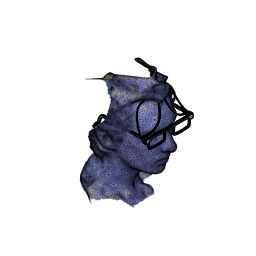
limelight_ (Autodesk Fusion 360 design; units mm, degrees)
Autodesk Fusion 360 part; units mm, degrees
note: some values were not read from the file. Set by a fixed rule: which sketch regions a step uses.
other "Base Mesh Feature1"
other "Scale1"
other "Modify1"
other "Scale2"
other "Modify2"
other "Scale3"
other "Modify3"
other "Modify4"
other "Base Mesh Feature2"
sketch "Sketch1" plane through (0, 0, 0) normal (1, 0, 0) x (0, 1, 0)
  line L0 (140.8479, 83.3353, 750) -> (440.7975, 83.3353, 750)
  line L1 (-324.1521, 83.3346, 750) -> (-324.1521, 110, 750)
  line L2 (-324.1521, 110, 750) -> (366, 110, 750)
  line L3 (440.7975, 83.3353, 750) -> (440.7975, 110, 750)
  line L4 (440.7975, 110, 750) -> (440.7975, 109, 750)
  arc A0 through (141.443, 83.3353, 750) (130.2389, 4.5049, 750) (140.8479, -74.4077, 750)
  arc A1 through (440.7975, -74.4077, 750) (453.6261, 4.4638, 750) (440.7975, 83.3353, 750)
  arc A2 through (140.8479, -74.4077, 750) (290.8227, -88.3663, 750) (440.7975, -74.4077, 750)
  line L5 (440.7975, 110, 750) -> (506.8968, 110, 750)
  line L6 (506.8968, 110, 750) -> (506.8968, 36.4474, 750)
  line L7 (506.8968, 36.4474, 750) -> (451.5624, 36.4474, 750)
  line L8 (-389.1, 110, 750) -> (-324.1521, 110, 750)
  line L9 (-389.1, 110.5472, 750) -> (-389.1, 36.4474, 750)
  line L10 (-334.8263, 36.5791, 750) -> (-389.1, 36.5791, 750)
  line L11 (366, 110, 750) -> (440.7975, 110, 750)
  line L12 (-324.1521, 83.3337, 750) -> (-324.1525, 83.3335, 750)
  line L13 (-24.2821, 83.3353, 750) -> (-324.2317, 83.3353, 750)
  arc A3 through (-324.2317, -74.4077, 750) (-337.0603, 4.4638, 750) (-324.2317, 83.3353, 750)
  arc A4 through (-24.2821, -74.4077, 750) (-174.2569, -88.3663, 750) (-324.2317, -74.4077, 750)
  arc A5 through (-24.8772, 83.3353, 750) (-13.6732, 4.5049, 750) (-24.2821, -74.4077, 750)
  line L14 (-24.8772, 83.3353, 750) -> (140.85, 83.3353, 750)
  arc A6 through (57.5187, -332.9413, 750) (68.7228, -411.7717, 750) (58.1138, -490.6843, 750)
  arc A7 through (58.1138, -490.6843, 750) (-91.861, -504.6429, 750) (-241.8358, -490.6843, 750)
  arc A8 through (-241.8358, -490.6843, 750) (-254.6644, -411.8128, 750) (-241.8358, -332.9413, 750)
  line L15 (58.1138, -332.9413, 750) -> (-241.8358, -332.9413, 750)
  line L16 (178.822, -332.9413, 750) -> (478.7716, -332.9413, 750)
  arc A9 through (179.4171, -332.9413, 750) (168.2131, -411.7717, 750) (178.822, -490.6843, 750)
  arc A10 through (178.822, -490.6843, 750) (328.7968, -504.6429, 750) (478.7716, -490.6843, 750)
  arc A11 through (478.7716, -490.6843, 750) (491.6002, -411.8128, 750) (478.7716, -332.9413, 750)
sketch "Sketch2" plane through (0, 0, 0) normal (1, 0, 0) x (0, 1, 0)
sketch "Sketch3" plane through (0, 0, 0) normal (0, 1, 0) x (1, 0, 0)
  line L0 (749.7214, -109.6566, 525) -> (-225, -109.6566, 525)
  line L1 (-225, -109.6566, 525) -> (-225, -75, 525)
  line L2 (-225, -75, 525) -> (750, -75, 525)
  line L3 (-225, -109.6566, 525) -> (-290.5465, -40.2965, 525)
  spline S0 degree 5 poles (-225, -109.6566, 525) (-229.9167, -109.8552, 525) (-239.5326, -109.7558, 525) (-253.3037, -108.1171, 525) (-270.3378, -102.903, 525) (-289.2972, -91.0605, 525) (-305.7958, -73.6023, 525) (-319.8038, -50.4603, 525) (-331.4877, -22.0144, 525) (-341.0832, 11.1976, 525) (-348.8293, 48.63, 525) (-353.7, 81.6023, 525) (-356.6609, 107.9114, 525) (-358.3321, 126.1414, 525) (-359.092, 135.4291, 525) knots 0 0 0 0 0 0 0.1 0.2 0.3 0.4 0.5 0.6 0.7 0.8 0.9 1 1 1 1 1 1
  spline S1 degree 5 poles (-225, -75, 525) (-228.9423, -74.8757, 525) (-236.6483, -74.1359, 525) (-247.6718, -71.5529, 525) (-261.2801, -65.1118, 525) (-276.384, -51.8165, 525) (-289.4959, -33.0418, 525) (-300.645, -8.8683, 525) (-309.999, 20.2425, 525) (-317.7601, 53.7351, 525) (-324.1234, 91.0724, 525) (-328.2167, 123.6855, 525) (-330.7671, 149.5743, 525) (-332.2403, 167.4582, 525) (-332.9201, 176.5564, 525) knots 0 0 0 0 0 0 0.1 0.2 0.3 0.4 0.5 0.6 0.7 0.8 0.9 1 1 1 1 1 1
  line L4 (-359.092, 135.4291, 525) -> (-332.9201, 176.5564, 525)
  line L5 (749.6084, -109.6566, 525) -> (749.6084, -75, 525)
  point P0 (-303.0094, -74.9766)
  point P1 (-283.692, -40.2965)
sketch "Sketch1 (curves 750 mm off its plane)" plane through (750, 0, 0) normal (1, 0, 0) x (0, 1, 0)
  line L0 (140.8479, 83.3353) -> (440.7975, 83.3353)
  line L1 (-324.1521, 83.3346) -> (-324.1521, 110)
  line L2 (-324.1521, 110) -> (366, 110)
  line L3 (440.7975, 83.3353) -> (440.7975, 110)
  line L4 (440.7975, 110) -> (440.7975, 109)
  arc A0 (141.443, 83.3353) -> (140.8479, -74.4077) centre (420.8756, 3.4085) ccw
  arc A1 (440.7975, -74.4077) -> (440.7975, 83.3353) centre (204.757, 4.4638) ccw
  arc A2 (140.8479, -74.4077) -> (440.7975, -74.4077) centre (290.8227, 724.3) ccw
  line L5 (440.7975, 110) -> (506.8968, 110)
  line L6 (506.8968, 110) -> (506.8968, 36.4474)
  line L7 (506.8968, 36.4474) -> (451.5624, 36.4474)
  line L8 (-389.1, 110) -> (-324.1521, 110)
  line L9 (-389.1, 110.5472) -> (-389.1, 36.4474)
  line L10 (-334.8263, 36.5791) -> (-389.1, 36.5791)
  line L11 (366, 110) -> (440.7975, 110)
  line L12 (-324.1521, 83.3337) -> (-324.1525, 83.3335)
  line L13 (-24.2821, 83.3353) -> (-324.2317, 83.3353)
  arc A3 (-324.2317, -74.4077) -> (-324.2317, 83.3353) centre (-88.1912, 4.4638) cw
  arc A4 (-24.2821, -74.4077) -> (-324.2317, -74.4077) centre (-174.2569, 724.3) cw
  arc A5 (-24.8772, 83.3353) -> (-24.2821, -74.4077) centre (-304.3099, 3.4085) cw
  line L14 (-24.8772, 83.3353) -> (140.85, 83.3353)
  arc A6 (57.5187, -332.9413) -> (58.1138, -490.6843) centre (-221.9139, -412.8681) cw
  arc A7 (58.1138, -490.6843) -> (-241.8358, -490.6843) centre (-91.861, 308.0234) cw
  arc A8 (-241.8358, -490.6843) -> (-241.8358, -332.9413) centre (-5.7953, -411.8128) cw
  line L15 (58.1138, -332.9413) -> (-241.8358, -332.9413)
  line L16 (178.822, -332.9413) -> (478.7716, -332.9413)
  arc A9 (179.4171, -332.9413) -> (178.822, -490.6843) centre (458.8497, -412.8681) ccw
  arc A10 (178.822, -490.6843) -> (478.7716, -490.6843) centre (328.7968, 308.0234) ccw
  arc A11 (478.7716, -490.6843) -> (478.7716, -332.9413) centre (242.7311, -411.8128) ccw
extrude "Extrude1" add sketch "Sketch1 (curves 750 mm off its plane)" against normal blind 25 contours L0 L1 L2 L3 L4 L11 L13 L14 | L0 A0 A1 A2 | L13 A3 A4 A5 | L3 L4 A1 L5 L6 L7 | L1 L8 L9 L10 L13 A3 makes body 1
sketch "Sketch3 (curves 525 mm off its plane)" plane through (0, 525, 0) normal (0, 1, 0) x (1, 0, 0)
  line L0 (749.7214, -109.6566) -> (-225, -109.6566)
  line L1 (-225, -109.6566) -> (-225, -75)
  line L2 (-225, -75) -> (750, -75)
  line L3 (-225, -109.6566) -> (-290.5465, -40.2965)
  spline S0 degree 5 poles (-225, -109.6566) (-229.9167, -109.8552) (-239.5326, -109.7558) (-253.3037, -108.1171) (-270.3378, -102.903) (-289.2972, -91.0605) (-305.7958, -73.6023) (-319.8038, -50.4603) (-331.4877, -22.0144) (-341.0832, 11.1976) (-348.8293, 48.63) (-353.7, 81.6023) (-356.6609, 107.9114) (-358.3321, 126.1414) (-359.092, 135.4291) knots 0 0 0 0 0 0 0.1 0.2 0.3 0.4 0.5 0.6 0.7 0.8 0.9 1 1 1 1 1 1
  spline S1 degree 5 poles (-225, -75) (-228.9423, -74.8757) (-236.6483, -74.1359) (-247.6718, -71.5529) (-261.2801, -65.1118) (-276.384, -51.8165) (-289.4959, -33.0418) (-300.645, -8.8683) (-309.999, 20.2425) (-317.7601, 53.7351) (-324.1234, 91.0724) (-328.2167, 123.6855) (-330.7671, 149.5743) (-332.2403, 167.4582) (-332.9201, 176.5564) knots 0 0 0 0 0 0 0.1 0.2 0.3 0.4 0.5 0.6 0.7 0.8 0.9 1 1 1 1 1 1
  line L4 (-359.092, 135.4291) -> (-332.9201, 176.5564)
  line L5 (749.6084, -109.6566) -> (749.6084, -75)
extrude "Extrude2" add sketch "Sketch3 (curves 525 mm off its plane)" along normal blind 20 separate body makes body 2
copy_body "CopyPasteBodies1" bodies 2 makes body 3
move_body "Move1" bodies 3 to x (1, 0, 0) y (0, 1, 0) z (0, 0, 1) at (0, -950, 0)
move_body "Move2" bodies 1 to x (1, 0, 0) y (0, 1, 0) z (0, 0, 1) at (50, 0, 0)
move_body "Move3" bodies 2 to x (1, 0, 0) y (0, 1, 0) z (0, 0, 1) at (100, 0, 0)
move_body "Move4" bodies 2 to x (1, 0, 0) y (0, 1, 0) z (0, 0, 1) at (-50, 0, 0)
extrude "Extrude3" add sketch "Sketch1 (curves 750 mm off its plane)" along normal blind 20 separate body contours A6 A7 A8 L15 | L16 A9 A10 A11 makes body 4 at (750, -108.8086, -389.6569) makes body 5 at (750, 345.7444, -389.6569)
scale "Scale1'" factor 0.9 about (770, 57.5187, -332.9413) bodies 4 5
move_body "Move5" bodies 4 to x (1, 0, 0) y (0, 1, 0) z (0, 0, 1) at (0, -100.648, 411.847)
move_body "Move6" bodies 5 to x (1, 0, 0) y (0, 1, 0) z (0, 0, 1) at (-50, -6.9412, 414.1607)
move_body "Move7" bodies 4 to x (1, 0, 0) y (0, 1, 0) z (0, 0, 1) at (-50, 0, 0)
move_body "Move8" bodies 5 to x (1, 0, 0) y (0, 1, 0) z (0, 0, 1) at (0, -0.8429, -2.0422)
extrude "Extrude4" cut 2 faces at (720, 309.1377, 28.1332) (720, -192.8239, 27.8617) along direction (1, 0, 0) blind 220 on bodies 4 5 bodies 1
other "Scale4"
other "Modify5"
other "Scale5"
other "Modify6"
other "Scale6"
other "Scale7"
scale "Scale2'" factor 0.2 about (-225, -405, 109.6566) bodies 3 1 2
move_body "Move9" bodies 3 1 2 to x (1, 0, 0) y (0, 1, 0) z (0, 0, 1) at (125, 283.3936, -86.4445)
scale "Scale3'" factor 0.7 about (-90, 68.3936, 23.2122) bodies 2 1 3
move_body "Move10" bodies 1 2 3 to x (1, 0, 0) y (0, 1, 0) z (0, 0, 1) at (40, -35, -5)
move_face "OffsetFaces1" offset -30 2 faces at (86.4452, 32.4603, 14.9776) (79.4452, -100.5397, 14.9776) on bodies 2 3
fillet "Fillet1" radius 2.25 2 edges at (84.75, -46.3059, -7.5568) (84.75, -23.1877, -7.5568) on bodies 1
fillet "Fillet2" radius 0.1 12 edges at (86.5, -1.4641, -9.5087) (86.5, -22.9109, -7.239) (86.5, -24.6634, 4.2315) (86.5, -44.8302, 4.2315) (86.5, -46.5826, -7.239) (86.5, -68.0294, -9.5087) (83, -68.0294, -9.5087) (83, -46.5826, -7.239) (83, -44.8302, 4.2315) (83, -24.6634, 4.2315) (83, -22.9109, -7.239) (83, -1.4641, -9.5087) on bodies 1
sketch "Sketch4" plane through (0, 0, 0) normal (1, 0, 0) x (0, 1, 0)
  line L0 (28.0614, 18.257, 83) -> (28.0614, 8, 83)
  line L1 (28.0614, 8, 83) -> (20.3595, 8, 83)
  arc A0 through (20.3595, 8, 83) (20.4148, 11.2668, 83) (19.1998, 14.2997, 83)
  arc A1 through (19.1998, 14.5242, 83) (19.1663, 14.4119, 83) (19.1998, 14.2997, 83)
  line L2 (19.1998, 14.5242, 83) -> (19.1998, 18.2279, 83)
  line L3 (19.1998, 18.2279, 83) -> (28.0614, 18.257, 83)
  line L4 (-88.4567, 18.1832, 82.9817) -> (-97.3183, 18.2123, 82.9817)
  line L5 (-88.4567, 14.4795, 82.9817) -> (-88.4567, 18.1832, 82.9817)
  arc A2 through (-89.6164, 7.9553, 82.9817) (-89.6717, 11.2221, 82.9817) (-88.4567, 14.255, 82.9817)
  line L6 (-97.3183, 7.9553, 82.9817) -> (-89.6164, 7.9553, 82.9817)
  line L7 (-97.3183, 18.2123, 82.9817) -> (-97.3183, 7.9553, 82.9817)
  line L8 (-88.4567, 14.4808, 82.9817) -> (-88.4567, 14.255, 82.9817)
sketch "Sketch4 (curves 82.9817 mm off its plane)" plane through (82.9817, 0, 0) normal (1, 0, 0) x (0, 1, 0)
  line L0 (-88.4567, 18.1832) -> (-97.3183, 18.2123)
  line L1 (-88.4567, 14.4795) -> (-88.4567, 18.1832)
  arc A0 (-89.6164, 7.9553) -> (-88.4567, 14.255) centre (-81.5439, 9.7258) cw
  line L2 (-97.3183, 7.9553) -> (-89.6164, 7.9553)
  line L3 (-97.3183, 18.2123) -> (-97.3183, 7.9553)
  line L4 (-88.4567, 14.4808) -> (-88.4567, 14.255)
extrude "Extrude5" add sketch "Sketch4 (curves 82.9817 mm off its plane)" against normal blind 8 separate body makes body 6
sketch "Sketch4 (curves 83 mm off its plane)" plane through (83, 0, 0) normal (1, 0, 0) x (0, 1, 0)
  line L0 (28.0614, 18.257) -> (28.0614, 8)
  line L1 (28.0614, 8) -> (20.3595, 8)
  arc A0 (20.3595, 8) -> (19.1998, 14.2997) centre (12.287, 9.7705) ccw
  arc A1 (19.1998, 14.5242) -> (19.1998, 14.2997) centre (19.3711, 14.4119) ccw
  line L2 (19.1998, 14.5242) -> (19.1998, 18.2279)
  line L3 (19.1998, 18.2279) -> (28.0614, 18.257)
extrude "Extrude6" add sketch "Sketch4 (curves 83 mm off its plane)" against normal blind 8 separate body makes body 7
sketch "Sketch5" plane through (0, 0, 0) normal (1, 0, 0) x (0, 1, 0)
  line L0 (27.0584, 11.8394, 75) -> (23.6584, 11.8394, 75)
  line L1 (23.6584, 11.8394, 75) -> (23.6584, 17.2394, 75)
  line L2 (23.6584, 17.2394, 75) -> (27.0584, 17.2394, 75)
  line L3 (27.0584, 17.2394, 75) -> (27.0584, 11.8394, 75)
  line L4 (27.0584, 11.8394, 75) -> (23.6584, 17.2394, 75) construction
  line L5 (23.6584, 11.8394, 75) -> (27.0584, 17.2394, 75) construction
  line L6 (-92.9416, 17.2394, 74.98) -> (-92.9416, 11.8394, 74.98)
  line L7 (-92.9416, 11.8394, 74.98) -> (-96.3416, 11.8394, 74.98)
  line L8 (-96.3416, 17.2394, 74.98) -> (-92.9416, 17.2394, 74.98)
  line L9 (-96.3416, 11.8394, 74.98) -> (-96.3416, 17.2394, 74.98)
  line L10 (-92.9416, 11.8394, 74.98) -> (-96.3416, 17.2394, 74.98) construction
  line L11 (-96.3416, 11.8394, 74.98) -> (-92.9416, 17.2394, 74.98) construction
  point P0 (25.3584, 14.5394)
  point P1 (-94.6416, 14.5394)
sketch "Sketch5 (curves 75 mm off its plane)" plane through (75, 0, 0) normal (1, 0, 0) x (0, 1, 0)
  line L0 (27.0584, 11.8394) -> (23.6584, 11.8394)
  line L1 (23.6584, 11.8394) -> (23.6584, 17.2394)
  line L2 (23.6584, 17.2394) -> (27.0584, 17.2394)
  line L3 (27.0584, 17.2394) -> (27.0584, 11.8394)
  line L4 (27.0584, 11.8394) -> (23.6584, 17.2394) construction
  line L5 (23.6584, 11.8394) -> (27.0584, 17.2394) construction
extrude "Extrude7" cut sketch "Sketch5 (curves 75 mm off its plane)" along normal blind 7 bodies 7
sketch "Sketch5 (curves 74.98 mm off its plane)" plane through (74.98, 0, 0) normal (1, 0, 0) x (0, 1, 0)
  line L0 (-92.9416, 17.2394) -> (-92.9416, 11.8394)
  line L1 (-92.9416, 11.8394) -> (-96.3416, 11.8394)
  line L2 (-96.3416, 17.2394) -> (-92.9416, 17.2394)
  line L3 (-96.3416, 11.8394) -> (-96.3416, 17.2394)
  line L4 (-92.9416, 11.8394) -> (-96.3416, 17.2394) construction
  line L5 (-96.3416, 11.8394) -> (-92.9416, 17.2394) construction
extrude "Extrude8" cut sketch "Sketch5 (curves 74.98 mm off its plane)" along normal blind 7 bodies 6
delete_face "DeleteFace1" 1 faces at (77.6667, 19.1945, 14.3081) on bodies 7
fillet "Fillet3" radius 0.25 12 edges at (74.9817, -97.3183, 13.0838) (74.9817, -92.8875, 18.1978) (74.9817, -88.4567, 16.2191) (74.9817, -89.6717, 11.2221) (74.9817, -93.4674, 7.9553) (78.9817, -88.4567, 14.255) (79, 19.1998, 14.2997) (75, 19.1998, 16.2638) (75, 20.4148, 11.2668) (75, 23.6306, 18.2425) (75, 28.0614, 13.1285) (75, 24.2105, 8) on bodies 6 7
fillet "Fillet4" radius 0.1 4 edges at (79.1067, -89.6164, 7.9553) (75.0383, -89.7295, 8.0469) (79.125, 20.3595, 8) (75.0566, 20.4725, 8.0916) on bodies 6 7
fillet "Fillet5" radius 0.15 4 edges at (79.1067, -88.4567, 18.1832) (75.0549, -88.5299, 18.1103) (79.125, 19.1998, 18.2279) (75.0732, 19.273, 18.155) on bodies 6 7
fillet "Fillet6" radius 0.5 8 edges at (-60.5275, 33.3936, 3.9291) (3.2226, 33.3936, 13.3602) (3.2226, 30.5936, 13.3602) (-60.5275, 30.5936, 3.9291) (-67.5275, -99.6064, 3.9291) (-3.7774, -99.6064, 13.3602) (-3.7774, -102.4064, 13.3602) (-67.5275, -102.4064, 3.9291) on bodies 2 3
move_body "Move11" bodies 2 to x (1, 0, 0) y (0, 1, 0) z (0, 0, 1) at (25, 0, 0)
move_body "Move12" bodies 3 to x (1, 0, 0) y (0, 1, 0) z (0, 0, 1) at (30, 0, 0)
move_body "Move13" bodies 1 7 6 to x (1, 0, 0) y (0, 1, 0) z (0, 0, 1) at (0, 10, 0)
sketch "Sketch6" plane through (0, 33.3936, 0) normal (0, 1, 0) x (-1, 0, 0)
  line L0 (-81.4452, 13.8602) -> (25.0079, 13.8602)
  spline S0 degree 3 poles (40.5566, -21.154) (40.2972, -17.824) (39.9613, -14.4995) (39.1496, -8.5924) (38.7212, -6.0065) (37.6122, -0.8835) (36.9383, 1.6625) (35.994, 4.1092) (35.5897, 5.1566) (35.1338, 6.1847) (33.7486, 8.7534) (32.6897, 10.2436) (30.2327, 12.3629) (28.9376, 13.0817) (26.7221, 13.7092) (25.8698, 13.8331) (25.0158, 13.86) (25.0131, 13.8601) (25.0105, 13.8602) (25.0079, 13.8602) knots -4.142023 -4.142023 -4.142023 -4.142023 -3.14001 -3.14001 -2.35323 -2.35323 -1.566445 -1.566445 -1.566445 -1.229621 -1.229621 -0.690703 -0.690703 -0.256348 -0.256348 0 0 0 0.000788 0.000788 0.000788 0.000788
  line L1 (40.5566, -21.154) -> (43.7729, -16.0998)
  spline S1 degree 5 poles (43.7729, -16.0998) (43.6665, -14.7996) (43.4325, -12.2473) (43.018, -8.5641) (42.3361, -3.948) (41.2516, 1.2926) (39.9083, 5.9423) (38.2725, 9.9247) (36.3114, 13.1646) (34.0016, 15.6087) (31.3473, 17.2667) (28.9625, 17.9966) (27.0346, 18.2261) (25.6883, 18.24) (25, 18.2122) knots -1 -1 -1 -1 -1 -1 -0.9 -0.8 -0.7 -0.6 -0.5 -0.4 -0.3 -0.2 -0.1 0 0 0 0 0 0
  line L2 (25, 18.2122) -> (-81.4452, 18.2122)
  line L3 (-81.4452, 18.2122) -> (-81.4452, 13.8602)
  spline S2 degree 5 poles (42.7082, -6.7221) (43.0306, -6.6571) (43.6683, -6.5541) (44.6034, -6.4806) (45.8069, -6.5473) (47.2345, -6.922) (48.5801, -7.6082) (49.8395, -8.6212) (51.0149, -9.9531) (52.1131, -11.5781) (53.1417, -13.4672) (53.9142, -15.1695) (54.4672, -16.5465) (54.8243, -17.5082) (55, -18) knots 0 0 0 0 0 0 0.1 0.2 0.3 0.4 0.5 0.6 0.7 0.8 0.9 1 1 1 1 1 1
  spline S3 degree 5 poles (42.988, -8.7008) (43.2023, -8.5839) (43.6304, -8.3839) (44.2715, -8.1857) (45.124, -8.1282) (46.1856, -8.4193) (47.243, -9.0924) (48.2962, -10.1488) (49.3454, -11.5605) (50.3911, -13.2902) (51.4337, -15.3007) (52.2656, -17.1101) (52.8883, -18.572) (53.303, -19.5925) (53.5102, -20.1142) knots 0 0 0 0 0 0 0.1 0.2 0.3 0.4 0.5 0.6 0.7 0.8 0.9 1 1 1 1 1 1
  line L4 (53.5102, -20.1142) -> (55, -18)
  circle A0 centre (55, -20) radius 2.1213
  point P0 (49, -8)
  point P1 (47, -9)
  constraint coincident S1 S2.start
  constraint coincident S1 S3.start
extrude "Extrude9" add sketch "Sketch6" against normal blind 3 separate body contours S1 S2 S3 A0 | S2 S3 L4 A0 | S2 S3 L4 A0 makes body 8
copy_body "CopyPasteBodies2" bodies 8 makes body 9
move_body "Move14" bodies 9 to x (1, 0, 0) y (0, 1, 0) z (0, 0, 1) at (0, -133, 0)
move_body "Move15" bodies 2 8 to x (1, 0, 0) y (0, 1, 0) z (0, 0, 1) at (0.8147, 3.352, -1.2314)
move_body "Move16" bodies 3 9 to x (1, 0, 0) y (0, 1, 0) z (0, 0, 1) at (-0.3292, 16.5, -0.9443)
sketch "Sketch7" plane through (0, 0, 16.9808) normal (0, 0, 1) x (-1, 0, 0)
  line L0 (24.1853, -33.9456) -> (-82.2599, -33.9456)
  line L1 (-82.2599, -33.9456) -> (-82.2599, -36.7456)
  line L2 (-82.2599, -36.7456) -> (24.1853, -36.7456)
  line L3 (24.1853, -36.7456) -> (24.1853, -33.9456)
  line L4 (-58.886, -33.9456) -> (-52.6505, -33.9456)
  line L5 (-52.6505, -33.9456) -> (-52.6505, -36.7456)
  line L6 (-52.6505, -36.7456) -> (-58.886, -36.7456)
  line L7 (-58.886, -36.7456) -> (-58.886, -33.9456)
  constraint horizontal L4
  constraint vertical L5
  constraint horizontal L6
  constraint vertical L7
  constraint coincident L2 L5.end
  constraint coincident L0 L4.start
sketch "Sketch8" plane through (0, 36.7456, 0) normal (0, 1, 0) x (-1, 0, 0)
  line L0 (-82.2599, 12.6288) -> (24.1931, 12.6288)
  spline S0 degree 3 poles (39.7418, -22.3854) (39.4825, -19.0554) (39.1466, -15.7309) (38.3348, -9.8238) (37.9065, -7.2379) (36.7974, -2.1149) (36.1236, 0.4311) (35.1792, 2.8778) (34.7749, 3.9252) (34.3191, 4.9533) (32.9339, 7.522) (31.875, 9.0122) (29.418, 11.1315) (28.1229, 11.8503) (25.9073, 12.4778) (25.0551, 12.6017) (24.201, 12.6286) (24.1984, 12.6287) (24.1958, 12.6288) (24.1931, 12.6288) knots -4.142023 -4.142023 -4.142023 -4.142023 -3.14001 -3.14001 -2.35323 -2.35323 -1.566445 -1.566445 -1.566445 -1.229621 -1.229621 -0.690703 -0.690703 -0.256348 -0.256348 0 0 0 0.000788 0.000788 0.000788 0.000788
  line L1 (39.7418, -22.3854) -> (42.9581, -17.3312)
  spline S1 degree 5 poles (42.9581, -17.3312) (42.8518, -16.031) (42.6178, -13.4787) (42.2033, -9.7955) (41.5214, -5.1794) (40.4369, 0.0612) (39.0935, 4.7109) (37.4578, 8.6933) (35.4967, 11.9332) (33.1869, 14.3773) (30.5326, 16.0353) (28.1478, 16.7652) (26.2198, 16.9947) (24.8736, 17.0086) (24.1853, 16.9808) knots -1 -1 -1 -1 -1 -1 -0.9 -0.8 -0.7 -0.6 -0.5 -0.4 -0.3 -0.2 -0.1 0 0 0 0 0 0
  line L2 (24.1853, 16.9808) -> (-82.2599, 16.9808)
  line L3 (-82.2599, 16.9808) -> (-82.2599, 12.6288)
  spline S2 degree 5 poles (-56, 19) (-56.5276, 20.0173) (-57.5618, 22.0263) (-59.0501, 24.9632) (-60.9065, 28.7234) (-62.9962, 33.1433) (-64.8263, 37.2476) (-66.359, 40.9905) (-67.5538, 44.3228) (-68.3753, 47.2013) (-68.8111, 49.611) (-68.8621, 51.1771) (-68.7404, 52.1573) (-68.5894, 52.7258) (-68.4965, 52.9889) knots 0 0 0 0 0 0 0.1 0.2 0.3 0.4 0.5 0.6 0.7 0.8 0.9 1 1 1 1 1 1
  point P0 (-68, 46)
sketch "Sketch9" plane through (0, 0, 0) normal (0, 1, 0) x (1, 0, 0)
sketch "Sketch10" plane through (0, 0, 0) normal (0, 1, 0) x (1, 0, 0)
  line L0 (82.2599, -16.9808, 33.9456) -> (-24.1853, -16.9808, 33.9456)
  spline S0 degree 5 poles (72.969, -16.9808, 33.9456) (73.5647, -17.0667, 32.6439) (74.7024, -17.3206, 30.035) (76.2488, -17.9472, 26.1054) (77.9845, -19.2826, 20.833) (79.5596, -21.8415, 14.2176) (80.4425, -25.3684, 7.683) (80.4927, -29.9429, 1.4345) (79.5156, -35.6029, -4.1261) (77.4814, -42.2931, -8.8382) (74.4249, -49.9323, -12.6534) (71.2128, -56.7382, -15.0044) (68.3962, -62.2082, -16.3897) (66.3404, -66.0146, -17.148) (65.268, -67.9578, -17.4859) knots 0 0 0 0 0 0 0.1 0.2 0.3 0.4 0.5 0.6 0.7 0.8 0.9 1 1 1 1 1 1
  line L1 (80.3514, -22.7518, 11.3742) -> (80.3514, -32.9272, -2.2709)
  spline S1 degree 5 poles (72.969, -16.9808, 33.9456) (73.5647, -17.0667, 32.6439) (74.7024, -17.3206, 30.035) (76.2488, -17.9472, 26.1054) (77.9845, -19.2826, 20.833) (79.5596, -21.8415, 14.2176) (80.4425, -25.3684, 7.683) (80.4927, -29.9429, 1.4345) (79.5156, -35.6029, -4.1261) (77.4814, -42.2931, -8.8382) (74.4249, -49.9323, -12.6534) (71.2128, -56.7382, -15.0044) (68.3962, -62.2082, -16.3897) (66.3404, -66.0146, -17.148) (65.268, -67.9578, -17.4859) knots 0 0 0 0 0 0 0.1 0.2 0.3 0.4 0.5 0.6 0.7 0.8 0.9 1 1 1 1 1 1
  line L2 (80.3514, -22.7518, 11.3742) -> (80.3514, -32.9272, -2.2709)
  spline S2 degree 5 poles (69.969, -16.9808, 36.9456) (70.5647, -17.0667, 35.6439) (71.7024, -17.3206, 33.035) (73.2488, -17.9472, 29.1054) (74.9845, -19.2826, 23.833) (76.5596, -21.8415, 17.2176) (77.4425, -25.3684, 10.683) (77.4927, -29.9429, 4.4345) (76.5156, -35.6029, -1.1261) (74.4814, -42.2931, -5.8382) (71.4249, -49.9323, -9.6534) (68.2128, -56.7382, -12.0044) (65.3962, -62.2082, -13.3897) (63.3404, -66.0146, -14.148) (62.268, -67.9578, -14.4859) knots 0 0 0 0 0 0 0.1 0.2 0.3 0.4 0.5 0.6 0.7 0.8 0.9 1 1 1 1 1 1
  line L3 (77.3514, -22.7518, 14.3742) -> (77.3514, -32.9272, 0.7291)
  line L4 (72.969, -16.9808, 33.9456) -> (69.969, -16.9808, 36.9456)
  line L5 (65.268, -67.9578, -17.4859) -> (62.268, -67.9578, -14.4859)
  spline S3 degree 5 poles (70.969, -16.9808, 33.9456) (71.5647, -17.0667, 32.6439) (72.7024, -17.3206, 30.035) (74.2488, -17.9472, 26.1054) (75.9845, -19.2826, 20.833) (77.5596, -21.8415, 14.2176) (78.4425, -25.3684, 7.683) (78.4927, -29.9429, 1.4345) (77.5156, -35.6029, -4.1261) (75.4814, -42.2931, -8.8382) (72.4249, -49.9323, -12.6534) (69.2128, -56.7382, -15.0044) (66.3962, -62.2082, -16.3897) (64.3404, -66.0146, -17.148) (63.268, -67.9578, -17.4859) knots 0 0 0 0 0 0 0.1 0.2 0.3 0.4 0.5 0.6 0.7 0.8 0.9 1 1 1 1 1 1
  line L6 (78.3514, -22.7518, 11.3742) -> (78.3514, -32.9272, -2.2709)
  point P0 (80.3514, -27.8395)
  point P1 (80.3514, -27.8395)
  point P2 (77.3514, -27.8395)
  point P3 (78.3514, -27.8395)
sketch "Sketch12" plane through (0, 36.7456, 0) normal (0, 1, 0) x (-1, 0, 0)
  line L0 (-82.2599, 12.6288) -> (24.1931, 12.6288)
  spline S0 degree 3 poles (39.7418, -22.3854) (39.4825, -19.0554) (39.1466, -15.7309) (38.3348, -9.8238) (37.9065, -7.2379) (36.7974, -2.1149) (36.1236, 0.4311) (35.1792, 2.8778) (34.7749, 3.9252) (34.3191, 4.9533) (32.9339, 7.522) (31.875, 9.0122) (29.418, 11.1315) (28.1229, 11.8503) (25.9073, 12.4778) (25.0551, 12.6017) (24.201, 12.6286) (24.1984, 12.6287) (24.1958, 12.6288) (24.1931, 12.6288) knots -4.142023 -4.142023 -4.142023 -4.142023 -3.14001 -3.14001 -2.35323 -2.35323 -1.566445 -1.566445 -1.566445 -1.229621 -1.229621 -0.690703 -0.690703 -0.256348 -0.256348 0 0 0 0.000788 0.000788 0.000788 0.000788
  line L1 (39.7418, -22.3854) -> (42.9581, -17.3312)
  spline S1 degree 5 poles (42.9581, -17.3312) (42.8518, -16.031) (42.6178, -13.4787) (42.2033, -9.7955) (41.5214, -5.1794) (40.4369, 0.0612) (39.0935, 4.7109) (37.4578, 8.6933) (35.4967, 11.9332) (33.1869, 14.3773) (30.5326, 16.0353) (28.1478, 16.7652) (26.2198, 16.9947) (24.8736, 17.0086) (24.1853, 16.9808) knots -1 -1 -1 -1 -1 -1 -0.9 -0.8 -0.7 -0.6 -0.5 -0.4 -0.3 -0.2 -0.1 0 0 0 0 0 0
  line L2 (24.1853, 16.9808) -> (-82.2599, 16.9808)
  line L3 (-82.2599, 16.9808) -> (-82.2599, 12.6288)
  line L4 (-72.9443, 16.9808) -> (-70, 16.9808)
  line L5 (-70, 16.9808) -> (-70, 18.5)
  line L6 (-70, 18.5) -> (-72.9443, 18.5)
  line L7 (-72.9443, 18.5) -> (-72.9443, 16.9808)
  constraint horizontal L4
  constraint vertical L5
  constraint horizontal L6
  constraint vertical L7
  constraint coincident L2 L4.start
sweep "Sweep2" add profiles "Sketch12" path "Sketch10" along S3 section 1 contours L2 L4 L5 L6 L7 separate body makes body 10
copy_body "CopyPasteBodies3" bodies 10 makes body 11
move_body "Move17" bodies 11 to x (1, 0, 0) y (0, 1, 0) z (0, 0, 1) at (0, -115, 0)
mirror "Mirror1" about plane through (0, 0, 0) normal (0, 1, 0) of bodies 11 makes body 12
move_body "Move18" bodies 12 to x (1, 0, 0) y (0, 1, 0) z (0, 0, 1) at (0, -165, 0)
sketch "Sketch13" plane through (0, 0, 0) normal (0, 0, 1) x (1, 0, 0)
  circle A0 centre (42, -1) radius 5
  circle A1 centre (46.984, -53.4308) radius 5.6072
extrude "Extrude10" add sketch "Sketch13" along normal blind 150 separate body makes body 13 at (52.5842, -53.7103, 100) makes body 14 at (46.9938, -1.2492, 100)
sketch "Sketch15" plane through (0, -85.9064, 0) normal (0, -1, 0) x (1, 0, 0)
  line L0 (-27.3371, 12.916) -> (79.1159, 12.916)
  line L1 (79.1159, 12.916) -> (79.1159, 17.2679)
  line L2 (79.1159, 17.2679) -> (-27.3292, 17.2679)
  spline S0 degree 5 poles (-27.3292, 17.2679) (-28.0176, 17.2957) (-29.3638, 17.2818) (-31.2917, 17.0524) (-33.6765, 16.3224) (-36.3308, 14.6645) (-38.6406, 12.2203) (-40.6018, 8.9804) (-42.2375, 4.998) (-43.5809, 0.3483) (-44.6653, -4.8922) (-45.3472, -9.5083) (-45.7617, -13.1916) (-45.9957, -15.7438) (-46.1021, -17.0441) knots 0 0 0 0 0 0 0.1 0.2 0.3 0.4 0.5 0.6 0.7 0.8 0.9 1 1 1 1 1 1
  line L3 (-46.1021, -17.0441) -> (-42.8858, -22.0983)
  spline S1 degree 3 poles (-27.3371, 12.916) (-27.3397, 12.9159) (-27.3424, 12.9158) (-27.345, 12.9157) (-28.1991, 12.8888) (-29.0513, 12.765) (-31.2669, 12.1374) (-32.5619, 11.4187) (-35.019, 9.2994) (-36.0779, 7.8092) (-37.463, 5.2405) (-37.9189, 4.2123) (-38.3232, 3.1649) (-39.2676, 0.7182) (-39.9414, -1.8277) (-41.0505, -6.9508) (-41.4788, -9.5366) (-42.2905, -15.4438) (-42.6264, -18.7682) (-42.8858, -22.0983) knots -0.000788 -0.000788 -0.000788 -0.000788 0 0 0 0.256348 0.256348 0.690703 0.690703 1.229621 1.229621 1.566445 1.566445 1.566445 2.35323 2.35323 3.14001 3.14001 4.142023 4.142023 4.142023 4.142023
  spline S2 degree 5 poles (66.4458, 17.2679, 0) (65.8897, 17.7184, -0.2345) (64.7875, 18.6442, -0.7012) (63.1644, 20.1078, -1.3945) (61.0609, 22.2095, -2.3054) (58.5354, 25.0879, -3.4214) (56.1207, 28.2131, -4.5158) (53.8284, 31.5715, -5.5908) (51.6759, 35.1356, -6.6507) (49.6881, 38.8577, -7.7022) (47.8952, 42.6723, -8.7556) (46.3279, 46.5044, -9.8256) (45.0127, 50.2752, -10.9321) (43.9677, 53.9093, -12.1018) (43.1971, 57.341, -13.3687) (42.686, 60.5215, -14.7758) (42.4063, 63.4164, -16.3702) (42.3244, 66.0029, -18.1975) (42.4064, 68.2681, -20.2967) (42.6255, 70.2065, -22.6943) (42.9652, 71.8188, -25.4016) (43.3257, 72.8506, -27.8173) (43.6442, 73.4809, -29.769) (43.8778, 73.8375, -31.132) (44, 74, -31.829) knots 0 0 0 0 0 0 0.05 0.1 0.15 0.2 0.25 0.3 0.35 0.4 0.45 0.5 0.55 0.6 0.65 0.7 0.75 0.8 0.85 0.9 0.95 1 1 1 1 1 1
  point P0 (53, 33)
  point P1 (44, 54)
  point P2 (42.3935, 67.3416)
sketch "Sketch16" plane through (0, -85.9064, 0) normal (0, -1, 0) x (1, 0, 0)
  line L0 (64.9842, 17.2675) -> (67.3698, 17.2675)
  line L1 (67.3698, 17.2675) -> (67.3698, 18.6988)
  line L2 (67.3698, 18.6988) -> (64.9842, 18.6988)
  line L3 (64.9842, 18.6988) -> (64.9842, 17.2675)
  constraint horizontal L0
  constraint vertical L1
  constraint horizontal L2
  constraint vertical L3
sweep "Sweep3" add profiles "Sketch16" path "Sketch15" along S2 section 1 separate body makes body 15
move_body "Move19" bodies 15 to x (1, 0, 0) y (0, 1, 0) z (0, 0, 1) at (4, 0, 0)
mirror "Mirror2" about plane through (0, 0, 0) normal (0, 1, 0) of bodies 15 makes body 16
move_body "Move20" bodies 16 to x (1, 0, 0) y (0, 1, 0) z (0, 0, 1) at (0, -50, 0)
hidden bodies 4 5 11 13 14
